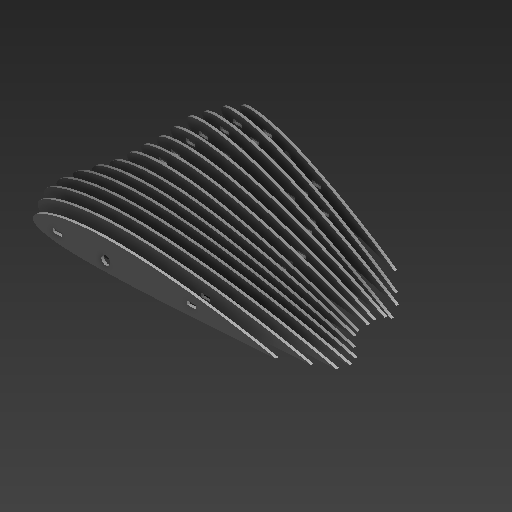
# Autodesk Inventor part: blade_all_sections
Saved by Autodesk Inventor 2027 (Build 310192000, 192)
## iProperties
Created: 2026-04-25
Part Number: blade_all_sections
Material: Generic
Document SubType Name: Modeling
Designer: charl
Density: 1 g/cm^3
Appearance: Default
Author: charl
Autodesk Inventor part; units mm, degrees
(part 1 of 6)
ref_plane "YZ Plane" through (0, 0, 0) normal (1, 0, 0) x (0, 1, 0)
ref_plane "XZ Plane" through (0, 0, 0) normal (0, 1, 0) x (-1, 0, 0)
ref_plane "XY Plane" through (0, 0, 0) normal (0, 0, 1) x (1, 0, 0)
sketch "Template_1mm" plane through (0, 0, 0) normal (0, 0, 1) x (1, 0, 0)
  spline S0 degree 4 poles (1, 0) (0.9999, 0) (0.9991, 0.0002) (0.9979, 0.0004) (0.9958, 0.0009) (0.9936, 0.0014) (0.991, 0.0019) (0.9878, 0.0026) (0.9842, 0.0033) (0.9801, 0.0042) (0.9755, 0.0051) (0.9705, 0.0062) (0.965, 0.0073) (0.959, 0.0085) (0.9526, 0.0098) (0.9457, 0.0112) (0.9384, 0.0126) (0.9307, 0.0141) (0.9226, 0.0157) (0.914, 0.0173) (0.905, 0.019) (0.8957, 0.0207) (0.8859, 0.0225) (0.8758, 0.0243) (0.8652, 0.0261) (0.8544, 0.028) (0.8431, 0.0299) (0.8315, 0.0319) (0.8196, 0.0338) (0.8074, 0.0358) (0.7949, 0.0378) (0.7821, 0.0398) (0.769, 0.0418) (0.7556, 0.0437) (0.742, 0.0457) (0.7281, 0.0477) (0.714, 0.0496) (0.6997, 0.0515) (0.6852, 0.0534) (0.6705, 0.0553) (0.6556, 0.0571) (0.6405, 0.0589) (0.6254, 0.0606) (0.6101, 0.0623) (0.5946, 0.0639) (0.5791, 0.0655) (0.5635, 0.067) (0.5478, 0.0684) (0.5321, 0.0698) (0.5164, 0.0711) (0.5006, 0.0723) (0.4848, 0.0735) (0.469, 0.0745) (0.4533, 0.0755) (0.4376, 0.0763) (0.4219, 0.0771) (0.4064, 0.0778) (0.3908, 0.0783) (0.3754, 0.0788) (0.36, 0.0791) (0.3448, 0.0792) (0.3297, 0.0792) (0.3148, 0.0791) (0.3001, 0.0788) (0.2855, 0.0784) (0.2712, 0.0778) (0.2571, 0.0771) (0.2433, 0.0763) (0.2298, 0.0753) (0.2165, 0.0742) (0.2035, 0.073) (0.1908, 0.0716) (0.1784, 0.0701) (0.1663, 0.0685) (0.1546, 0.0668) (0.1433, 0.065) (0.1323, 0.0631) (0.1217, 0.061) (0.1114, 0.0589) (0.1016, 0.0567) (0.0922, 0.0544) (0.0832, 0.052) (0.0746, 0.0496) (0.0665, 0.0471) (0.0588, 0.0445) (0.0515, 0.0419) (0.0447, 0.0393) (0.0384, 0.0366) (0.0325, 0.0338) (0.0271, 0.0311) (0.0222, 0.0283) (0.0178, 0.0255) (0.0138, 0.0227) (0.0103, 0.0199) (0.0074, 0.0171) (0.0049, 0.0142) (0.0029, 0.0114) (0.0014, 0.0085) (0.0004, 0.0057) (-0.0001, 0.0028) (-0.0001, 0) (0.0004, -0.0028) (0.0015, -0.0055) (0.003, -0.0081) (0.005, -0.0106) (0.0075, -0.013) (0.0105, -0.0153) (0.014, -0.0175) (0.0179, -0.0196) (0.0222, -0.0216) (0.0271, -0.0235) (0.0323, -0.0254) (0.0381, -0.0271) (0.0442, -0.0287) (0.0508, -0.0303) (0.0579, -0.0317) (0.0653, -0.0331) (0.0732, -0.0343) (0.0815, -0.0355) (0.0901, -0.0366) (0.0992, -0.0376) (0.1086, -0.0384) (0.1184, -0.0392) (0.1286, -0.0399) (0.1391, -0.0405) (0.15, -0.041) (0.1612, -0.0415) (0.1727, -0.0418) (0.1845, -0.0421) (0.1966, -0.0423) (0.209, -0.0424) (0.2217, -0.0424) (0.2347, -0.0423) (0.2479, -0.0422) (0.2613, -0.0421) (0.275, -0.0418) (0.2889, -0.0415) (0.303, -0.0412) (0.3173, -0.0408) (0.3318, -0.0404) (0.3464, -0.0399) (0.3612, -0.0394) (0.3761, -0.0389) (0.3911, -0.0383) (0.4063, -0.0378) (0.4217, -0.0371) (0.4371, -0.0365) (0.4526, -0.0358) (0.4682, -0.035) (0.4838, -0.0342) (0.4994, -0.0334) (0.515, -0.0326) (0.5306, -0.0317) (0.5462, -0.0308) (0.5618, -0.0299) (0.5772, -0.029) (0.5927, -0.0281) (0.608, -0.0271) (0.6232, -0.0262) (0.6383, -0.0252) (0.6533, -0.0243) (0.6681, -0.0233) (0.6828, -0.0224) (0.6973, -0.0214) (0.7116, -0.0205) (0.7257, -0.0195) (0.7395, -0.0186) (0.7532, -0.0177) (0.7666, -0.0168) (0.7797, -0.0159) (0.7926, -0.015) (0.8052, -0.0141) (0.8175, -0.0133) (0.8294, -0.0125) (0.8411, -0.0117) (0.8524, -0.0109) (0.8634, -0.0101) (0.874, -0.0093) (0.8842, -0.0086) (0.8941, -0.0079) (0.9036, -0.0072) (0.9126, -0.0065) (0.9213, -0.0059) (0.9296, -0.0053) (0.9374, -0.0047) (0.9448, -0.0042) (0.9518, -0.0037) (0.9583, -0.0032) (0.9643, -0.0027) (0.9699, -0.0023) (0.9751, -0.0019) (0.9797, -0.0016) (0.9839, -0.0012) (0.9876, -0.001) (0.9908, -0.0007) (0.9935, -0.0005) (0.9957, -0.0003) (0.9979, -0.0002) (0.9991, -0.0001) (0.9998, 0) (1, 0) knots 0 0 0 0 0 0.003306 0.005253 0.00752 0.010062 0.01285 0.015861 0.019079 0.022488 0.026078 0.029837 0.033757 0.037828 0.042045 0.046398 0.050884 0.055494 0.060224 0.065069 0.070023 0.075082 0.080241 0.085495 0.090841 0.096274 0.101791 0.107386 0.113057 0.118799 0.124609 0.130484 0.136419 0.142412 0.148458 0.154554 0.160697 0.166884 0.17311 0.179374 0.185671 0.191998 0.198352 0.20473 0.211128 0.217543 0.223972 0.230412 0.23686 0.243312 0.249765 0.256217 0.262663 0.2691 0.275526 0.281941 0.288345 0.294734 0.301105 0.307451 0.313767 0.320049 0.326294 0.332498 0.338659 0.344773 0.350837 0.356848 0.362801 0.368695 0.374525 0.380288 0.38598 0.391599 0.39714 0.4026 0.407976 0.413263 0.418458 0.423557 0.428556 0.433452 0.438241 0.442917 0.447478 0.451919 0.456236 0.460425 0.464482 0.468403 0.472185 0.475825 0.479322 0.482675 0.485889 0.48897 0.49193 0.494788 0.497572 0.50031 0.503032 0.505769 0.508552 0.511409 0.514365 0.517441 0.520647 0.523991 0.527474 0.531098 0.534861 0.538758 0.542789 0.546947 0.551231 0.555634 0.560154 0.564786 0.569527 0.574371 0.579315 0.584356 0.58949 0.594712 0.60002 0.605409 0.610877 0.61642 0.622034 0.627716 0.633463 0.639271 0.645138 0.651061 0.657035 0.663059 0.669128 0.675241 0.681393 0.687582 0.693804 0.700057 0.706341 0.712655 0.718998 0.725365 0.731751 0.738149 0.744556 0.750969 0.757385 0.7638 0.770211 0.776616 0.783011 0.789393 0.795759 0.802106 0.808429 0.814727 0.820996 0.827232 0.833433 0.839595 0.845714 0.851788 0.857813 0.863785 0.869702 0.875558 0.881352 0.887078 0.892735 0.898316 0.90382 0.909242 0.914577 0.919822 0.924972 0.930023 0.93497 0.939808 0.944533 0.949139 0.95362 0.95797 0.962183 0.966252 0.970169 0.973927 0.977515 0.980924 0.984141 0.987151 0.989939 0.99248 0.994747 0.996694 1 1 1 1 1
  point P0 (0, 0)
  point P1 (0.999, 0.0002)
  point P2 (0.9978, 0.0005)
  point P3 (0.9961, 0.0008)
  point P4 (0.9939, 0.0013)
  point P5 (0.9912, 0.0019)
  point P6 (0.9881, 0.0025)
  point P7 (0.9844, 0.0033)
  point P8 (0.9803, 0.0041)
  point P9 (0.9758, 0.0051)
  point P10 (0.9707, 0.0061)
  point P11 (0.9652, 0.0073)
  point P12 (0.9592, 0.0085)
  point P13 (0.9528, 0.0097)
  point P14 (0.946, 0.0111)
  point P15 (0.9387, 0.0125)
  point P16 (0.9309, 0.014)
  point P17 (0.9228, 0.0156)
  point P18 (0.9142, 0.0172)
  point P19 (0.9052, 0.0189)
  point P20 (0.8959, 0.0206)
  point P21 (0.8861, 0.0224)
  point P22 (0.8759, 0.0242)
  point P23 (0.8654, 0.0261)
  point P24 (0.8545, 0.028)
  point P25 (0.8433, 0.0299)
  point P26 (0.8317, 0.0318)
  point P27 (0.8198, 0.0338)
  point P28 (0.8076, 0.0358)
  point P29 (0.795, 0.0378)
  point P30 (0.7822, 0.0397)
  point P31 (0.7691, 0.0417)
  point P32 (0.7557, 0.0437)
  point P33 (0.7421, 0.0457)
  point P34 (0.7282, 0.0476)
  point P35 (0.7141, 0.0496)
  point P36 (0.6998, 0.0515)
  point P37 (0.6853, 0.0534)
  point P38 (0.6705, 0.0553)
  point P39 (0.6557, 0.0571)
  point P40 (0.6406, 0.0589)
  point P41 (0.6254, 0.0606)
  point P42 (0.6101, 0.0623)
  point P43 (0.5947, 0.0639)
  point P44 (0.5792, 0.0655)
  point P45 (0.5635, 0.067)
  point P46 (0.5479, 0.0684)
  point P47 (0.5321, 0.0698)
  point P48 (0.5164, 0.0711)
  point P49 (0.5006, 0.0723)
  point P50 (0.4848, 0.0734)
  point P51 (0.469, 0.0745)
  point P52 (0.4533, 0.0754)
  point P53 (0.4376, 0.0763)
  point P54 (0.4219, 0.0771)
  point P55 (0.4064, 0.0778)
  point P56 (0.3908, 0.0783)
  point P57 (0.3753, 0.0787)
  point P58 (0.3599, 0.079)
  point P59 (0.3447, 0.0792)
  point P60 (0.3296, 0.0792)
  point P61 (0.3147, 0.0791)
  point P62 (0.2999, 0.0788)
  point P63 (0.2854, 0.0784)
  point P64 (0.2711, 0.0778)
  point P65 (0.257, 0.0771)
  point P66 (0.2432, 0.0763)
  point P67 (0.2296, 0.0753)
  point P68 (0.2163, 0.0742)
  point P69 (0.2033, 0.0729)
  point P70 (0.1906, 0.0716)
  point P71 (0.1782, 0.0701)
  point P72 (0.1662, 0.0685)
  point P73 (0.1544, 0.0668)
  point P74 (0.1431, 0.0649)
  point P75 (0.1321, 0.063)
  point P76 (0.1215, 0.061)
  point P77 (0.1112, 0.0588)
  point P78 (0.1014, 0.0566)
  point P79 (0.092, 0.0543)
  point P80 (0.083, 0.052)
  point P81 (0.0744, 0.0495)
  point P82 (0.0663, 0.047)
  point P83 (0.0586, 0.0444)
  point P84 (0.0513, 0.0418)
  point P85 (0.0445, 0.0391)
  point P86 (0.0382, 0.0364)
  point P87 (0.0323, 0.0337)
  point P88 (0.027, 0.0309)
  point P89 (0.0221, 0.0282)
  point P90 (0.0176, 0.0253)
  point P91 (0.0137, 0.0225)
  point P92 (0.0102, 0.0197)
  point P93 (0.0073, 0.0169)
  point P94 (0.0048, 0.014)
  point P95 (0.0029, 0.0112)
  point P96 (0.0014, 0.0084)
  point P97 (0.0004, 0.0056)
  point P98 (0, 0.0028)
  point P99 (0, 0)
  point P100 (0.0005, -0.0027)
  point P101 (0.0015, -0.0054)
  point P102 (0.003, -0.008)
  point P103 (0.005, -0.0104)
  point P104 (0.0075, -0.0128)
  point P105 (0.0104, -0.0151)
  point P106 (0.0138, -0.0173)
  point P107 (0.0177, -0.0195)
  point P108 (0.0221, -0.0215)
  point P109 (0.0269, -0.0234)
  point P110 (0.0322, -0.0252)
  point P111 (0.0379, -0.027)
  point P112 (0.044, -0.0286)
  point P113 (0.0506, -0.0302)
  point P114 (0.0577, -0.0317)
  point P115 (0.0651, -0.033)
  point P116 (0.073, -0.0343)
  point P117 (0.0813, -0.0355)
  point P118 (0.0899, -0.0365)
  point P119 (0.099, -0.0375)
  point P120 (0.1084, -0.0384)
  point P121 (0.1182, -0.0392)
  point P122 (0.1284, -0.0399)
  point P123 (0.1389, -0.0405)
  point P124 (0.1498, -0.041)
  point P125 (0.161, -0.0414)
  point P126 (0.1725, -0.0418)
  point P127 (0.1844, -0.0421)
  point P128 (0.1965, -0.0422)
  point P129 (0.2089, -0.0423)
  point P130 (0.2216, -0.0424)
  point P131 (0.2346, -0.0423)
  point P132 (0.2478, -0.0422)
  point P133 (0.2612, -0.0421)
  point P134 (0.2749, -0.0418)
  point P135 (0.2888, -0.0415)
  point P136 (0.3029, -0.0412)
  point P137 (0.3172, -0.0408)
  point P138 (0.3317, -0.0404)
  point P139 (0.3463, -0.0399)
  point P140 (0.3611, -0.0394)
  point P141 (0.376, -0.0389)
  point P142 (0.3911, -0.0383)
  point P143 (0.4063, -0.0378)
  point P144 (0.4216, -0.0371)
  point P145 (0.4371, -0.0365)
  point P146 (0.4526, -0.0358)
  point P147 (0.4682, -0.035)
  point P148 (0.4838, -0.0342)
  point P149 (0.4994, -0.0334)
  point P150 (0.515, -0.0326)
  point P151 (0.5307, -0.0317)
  point P152 (0.5462, -0.0308)
  point P153 (0.5618, -0.0299)
  point P154 (0.5773, -0.029)
  point P155 (0.5927, -0.0281)
  point P156 (0.608, -0.0271)
  point P157 (0.6233, -0.0262)
  point P158 (0.6384, -0.0252)
  point P159 (0.6534, -0.0243)
  point P160 (0.6682, -0.0233)
  point P161 (0.6829, -0.0224)
  point P162 (0.6974, -0.0214)
  point P163 (0.7117, -0.0205)
  point P164 (0.7258, -0.0195)
  point P165 (0.7397, -0.0186)
  point P166 (0.7533, -0.0177)
  point P167 (0.7667, -0.0168)
  point P168 (0.7799, -0.0159)
  point P169 (0.7927, -0.015)
  point P170 (0.8053, -0.0141)
  point P171 (0.8176, -0.0133)
  point P172 (0.8296, -0.0125)
  point P173 (0.8413, -0.0116)
  point P174 (0.8526, -0.0108)
  point P175 (0.8636, -0.0101)
  point P176 (0.8742, -0.0093)
  point P177 (0.8844, -0.0086)
  point P178 (0.8943, -0.0079)
  point P179 (0.9038, -0.0072)
  point P180 (0.9129, -0.0065)
  point P181 (0.9215, -0.0059)
  point P182 (0.9298, -0.0053)
  point P183 (0.9376, -0.0047)
  point P184 (0.945, -0.0042)
  point P185 (0.952, -0.0037)
  point P186 (0.9585, -0.0032)
  point P187 (0.9646, -0.0027)
  point P188 (0.9702, -0.0023)
  point P189 (0.9753, -0.0019)
  point P190 (0.98, -0.0015)
  point P191 (0.9841, -0.0012)
  point P192 (0.9878, -0.0009)
  point P193 (0.9911, -0.0007)
  point P194 (0.9938, -0.0005)
  point P195 (0.996, -0.0003)
  point P196 (0.9978, -0.0002)
  point P197 (0.999, -0.0001)
  point P198 (0.9998, 0)
  constraints: 201 other
sketch "S01_282p7" plane through (0, 0, 0) normal (0, 0, 1) x (1, 0, 0)
  spline S0 degree 4 poles (197.89, 0) (197.8478, 0.0089) (197.6412, 0.0535) (197.2945, 0.127) (196.7094, 0.2515) (196.0938, 0.3827) (195.3375, 0.5419) (194.4468, 0.7301) (193.42, 0.9446) (192.2596, 1.1868) (190.9662, 1.454) (189.5407, 1.7472) (187.9852, 2.0644) (186.3002, 2.405) (184.4884, 2.7686) (182.5503, 3.1528) (180.4886, 3.5578) (178.305, 3.9817) (176.0014, 4.4244) (173.5799, 4.8834) (171.0432, 5.3581) (168.3934, 5.8471) (165.6328, 6.3494) (162.7648, 6.8637) (159.791, 7.3884) (156.7155, 7.9219) (153.54, 8.464) (150.2688, 9.0122) (146.9036, 9.5662) (143.4493, 10.1234) (139.9076, 10.6839) (136.2831, 11.2451) (132.5788, 11.8067) (128.7985, 12.3666) (124.9455, 12.924) (121.0243, 13.4777) (117.0377, 14.0257) (112.9904, 14.5674) (108.8863, 15.1011) (104.729, 15.6259) (100.5229, 16.1401) (96.2719, 16.6428) (91.9805, 17.1328) (87.6529, 17.6088) (83.2929, 18.069) (78.9059, 18.5129) (74.4948, 18.9397) (70.0653, 19.3466) (65.6209, 19.7344) (61.1668, 20.1005) (56.7065, 20.4449) (52.2457, 20.7659) (47.7877, 21.0617) (43.3377, 21.3337) (38.8997, 21.5782) (34.4748, 21.7965) (30.0745, 21.9858) (25.679, 22.1479) (21.302, 22.268) (16.9599, 22.3503) (12.6537, 22.3924) (8.3912, 22.3942) (4.1763, 22.3569) (0.0143, 22.2781) (-4.0915, 22.161) (-8.1355, 22.0027) (-12.1145, 21.806) (-16.0234, 21.5697) (-19.8589, 21.2958) (-23.6162, 20.9836) (-27.292, 20.6351) (-30.8818, 20.2504) (-34.3822, 19.8314) (-37.7896, 19.378) (-41.1001, 18.8929) (-44.3103, 18.3764) (-47.4177, 17.8306) (-50.4179, 17.2562) (-53.3089, 16.6561) (-56.0871, 16.0307) (-58.7501, 15.3815) (-61.2951, 14.7119) (-63.7196, 14.0219) (-66.0212, 13.3139) (-68.1983, 12.5902) (-70.248, 11.8516) (-72.169, 11.1005) (-73.9594, 10.3386) (-75.6179, 9.5672) (-77.1424, 8.7878) (-78.5328, 8.0024) (-79.7874, 7.2122) (-80.905, 6.4176) (-81.8865, 5.6212) (-82.7292, 4.8217) (-83.4343, 4.0206) (-84.0005, 3.2181) (-84.4265, 2.4131) (-84.7091, 1.6061) (-84.8481, 0.8003) (-84.8395, -0.0029) (-84.6887, -0.7919) (-84.3938, -1.5543) (-83.9585, -2.2892) (-83.3855, -2.9949) (-82.6774, -3.672) (-81.836, -4.3207) (-80.8623, -4.9429) (-79.7576, -5.5386) (-78.5226, -6.1081) (-77.1584, -6.6512) (-75.6665, -7.1679) (-74.048, -7.6582) (-72.3049, -8.1218) (-70.4387, -8.559) (-68.4516, -8.9688) (-66.3451, -9.3525) (-64.122, -9.7084) (-61.7838, -10.0379) (-59.3335, -10.3407) (-56.7729, -10.6165) (-54.1052, -10.8651) (-51.3323, -11.0888) (-48.4575, -11.2848) (-45.4833, -11.4565) (-42.4121, -11.602) (-39.2476, -11.7234) (-35.9922, -11.8211) (-32.6493, -11.8942) (-29.2217, -11.9463) (-25.7127, -11.9747) (-22.1257, -11.9838) (-18.464, -11.9717) (-14.7302, -11.941) (-10.929, -11.8928) (-7.0625, -11.8268) (-3.1355, -11.7458) (0.8493, -11.6499) (4.888, -11.5404) (8.977, -11.4191) (13.1124, -11.2874) (17.2906, -11.1451) (21.5102, -10.9956) (25.7647, -10.837) (30.0612, -10.676) (34.4055, -10.4993) (38.7678, -10.3113) (43.1533, -10.1102) (47.5518, -9.8987) (51.9606, -9.6775) (56.375, -9.4478) (60.7901, -9.2098) (65.2023, -8.9656) (69.607, -8.7144) (74.0002, -8.4593) (78.3772, -8.1988) (82.734, -7.936) (87.066, -7.6701) (91.3697, -7.4015) (95.6399, -7.1328) (99.8729, -6.8629) (104.0645, -6.5924) (108.2108, -6.3235) (112.3068, -6.0547) (116.3497, -5.7881) (120.3344, -5.5234) (124.2575, -5.2608) (128.1148, -5.0011) (131.9031, -4.7449) (135.6174, -4.4924) (139.255, -4.2434) (142.812, -3.9985) (146.2846, -3.759) (149.6692, -3.5233) (152.963, -3.2936) (156.162, -3.0687) (159.2633, -2.8504) (162.2636, -2.637) (165.1601, -2.4307) (167.9493, -2.2306) (170.6291, -2.0375) (173.1959, -1.851) (175.648, -1.6728) (177.982, -1.5013) (180.196, -1.3384) (182.2877, -1.1837) (184.2548, -1.0368) (186.0952, -0.8993) (187.8074, -0.7709) (189.389, -0.6512) (190.8386, -0.5416) (192.1549, -0.4409) (193.336, -0.3512) (194.3812, -0.2707) (195.2888, -0.201) (196.0589, -0.1419) (196.6867, -0.0929) (197.2832, -0.0475) (197.6364, -0.0194) (197.8469, -0.0032) (197.89, 0) knots 0 0 0 0 0 0.003306 0.005253 0.00752 0.010062 0.01285 0.015861 0.019079 0.022488 0.026078 0.029837 0.033757 0.037828 0.042045 0.046398 0.050884 0.055494 0.060224 0.065069 0.070023 0.075082 0.080241 0.085495 0.090841 0.096274 0.101791 0.107386 0.113057 0.118799 0.124609 0.130484 0.136419 0.142412 0.148458 0.154554 0.160697 0.166884 0.17311 0.179374 0.185671 0.191998 0.198352 0.20473 0.211128 0.217543 0.223972 0.230412 0.23686 0.243312 0.249765 0.256217 0.262663 0.2691 0.275526 0.281941 0.288345 0.294734 0.301105 0.307451 0.313767 0.320049 0.326294 0.332498 0.338659 0.344773 0.350837 0.356848 0.362801 0.368695 0.374525 0.380288 0.38598 0.391599 0.39714 0.4026 0.407976 0.413263 0.418458 0.423557 0.428556 0.433452 0.438241 0.442917 0.447478 0.451919 0.456236 0.460425 0.464482 0.468403 0.472185 0.475825 0.479322 0.482675 0.485889 0.48897 0.49193 0.494788 0.497572 0.50031 0.503032 0.505769 0.508552 0.511409 0.514365 0.517441 0.520647 0.523991 0.527474 0.531098 0.534861 0.538758 0.542789 0.546947 0.551231 0.555634 0.560154 0.564786 0.569527 0.574371 0.579315 0.584356 0.58949 0.594712 0.60002 0.605409 0.610877 0.61642 0.622034 0.627716 0.633463 0.639271 0.645138 0.651061 0.657035 0.663059 0.669128 0.675241 0.681393 0.687582 0.693804 0.700057 0.706341 0.712655 0.718998 0.725365 0.731751 0.738149 0.744556 0.750969 0.757385 0.7638 0.770211 0.776616 0.783011 0.789393 0.795759 0.802106 0.808429 0.814727 0.820996 0.827232 0.833433 0.839595 0.845714 0.851788 0.857813 0.863785 0.869702 0.875558 0.881352 0.887078 0.892735 0.898316 0.90382 0.909242 0.914577 0.919822 0.924972 0.930023 0.93497 0.939808 0.944533 0.949139 0.95362 0.95797 0.962183 0.966252 0.970169 0.973927 0.977515 0.980924 0.984141 0.987151 0.989939 0.99248 0.994747 0.996694 1 1 1 1 1
  circle A0 centre (0, 0) radius 5.15
  line L0 (-51.44, -2.1) -> (-61.64, -2.1)
  line L1 (-61.64, -2.1) -> (-61.64, 2.1)
  line L2 (-61.64, 2.1) -> (-51.44, 2.1)
  line L3 (-51.44, 2.1) -> (-51.44, -2.1)
  line L4 (-51.44, -2.1) -> (-61.64, 2.1) construction
  line L5 (-61.64, -2.1) -> (-51.44, 2.1) construction
  line L6 (105.1, 7.1) -> (94.9, 7.1)
  line L7 (94.9, 7.1) -> (94.9, 2.9)
  line L8 (94.9, 2.9) -> (105.1, 2.9)
  line L9 (105.1, 2.9) -> (105.1, 7.1)
  line L10 (105.1, 7.1) -> (94.9, 2.9) construction
  line L11 (94.9, 7.1) -> (105.1, 2.9) construction
  point P0 (197.6138, 0.0591)
  point P1 (197.2686, 0.1326)
  point P2 (196.7861, 0.2352)
  point P3 (196.1664, 0.3669)
  point P4 (195.4102, 0.5267)
  point P5 (194.518, 0.7147)
  point P6 (193.4906, 0.9298)
  point P7 (192.3293, 1.1718)
  point P8 (191.0351, 1.4395)
  point P9 (189.6089, 1.7327)
  point P10 (188.0523, 2.0501)
  point P11 (186.3666, 2.3911)
  point P12 (184.5536, 2.7546)
  point P13 (182.6146, 3.1394)
  point P14 (180.5517, 3.5445)
  point P15 (178.367, 3.9688)
  point P16 (176.0622, 4.4115)
  point P17 (173.6394, 4.8709)
  point P18 (171.1013, 5.3459)
  point P19 (168.4502, 5.8352)
  point P20 (165.6882, 6.3379)
  point P21 (162.8185, 6.8524)
  point P22 (159.8434, 7.3773)
  point P23 (156.7662, 7.9114)
  point P24 (153.5892, 8.4536)
  point P25 (150.3161, 9.0023)
  point P26 (146.9494, 9.5564)
  point P27 (143.4931, 10.1142)
  point P28 (139.9498, 10.6748)
  point P29 (136.3233, 11.2365)
  point P30 (132.6171, 11.7982)
  point P31 (128.8349, 12.3585)
  point P32 (124.98, 12.9163)
  point P33 (121.0567, 13.4701)
  point P34 (117.068, 14.0185)
  point P35 (113.0187, 14.5605)
  point P36 (108.9124, 15.0945)
  point P37 (104.7531, 15.6195)
  point P38 (100.5448, 16.134)
  point P39 (96.2916, 16.6369)
  point P40 (91.9979, 17.1271)
  point P41 (87.6681, 17.6032)
  point P42 (83.306, 18.0637)
  point P43 (78.9166, 18.5078)
  point P44 (74.5033, 18.9344)
  point P45 (70.0714, 19.3418)
  point P46 (65.6248, 19.7294)
  point P47 (61.1684, 20.0957)
  point P48 (56.7059, 20.4401)
  point P49 (52.2427, 20.7609)
  point P50 (47.7825, 21.0572)
  point P51 (43.3303, 21.3286)
  point P52 (38.8902, 21.5734)
  point P53 (34.4671, 21.7911)
  point P54 (30.0651, 21.9805)
  point P55 (25.668, 22.1397)
  point P56 (21.2865, 22.2606)
  point P57 (16.9394, 22.3423)
  point P58 (12.631, 22.3842)
  point P59 (8.3662, 22.3859)
  point P60 (4.1495, 22.3477)
  point P61 (-0.0147, 22.2691)
  point P62 (-4.1223, 22.151)
  point P63 (-8.1683, 21.9926)
  point P64 (-12.149, 21.795)
  point P65 (-16.0599, 21.5584)
  point P66 (-19.897, 21.2836)
  point P67 (-23.6561, 20.971)
  point P68 (-27.3334, 20.6216)
  point P69 (-30.9248, 20.2362)
  point P70 (-34.4266, 19.8161)
  point P71 (-37.8354, 19.3621)
  point P72 (-41.1473, 18.8759)
  point P73 (-44.3587, 18.3585)
  point P74 (-47.467, 17.8115)
  point P75 (-50.4685, 17.2362)
  point P76 (-53.3602, 16.6346)
  point P77 (-56.1391, 16.0079)
  point P78 (-58.8027, 15.3577)
  point P79 (-61.3482, 14.6863)
  point P80 (-63.7729, 13.9948)
  point P81 (-66.0746, 13.2852)
  point P82 (-68.2514, 12.5595)
  point P83 (-70.3007, 11.8191)
  point P84 (-72.2208, 11.066)
  point P85 (-74.01, 10.3019)
  point P86 (-75.6666, 9.5281)
  point P87 (-77.189, 8.7465)
  point P88 (-78.5762, 7.9586)
  point P89 (-79.8266, 7.1659)
  point P90 (-80.9393, 6.3695)
  point P91 (-81.9137, 5.5712)
  point P92 (-82.7486, 4.7714)
  point P93 (-83.4437, 3.9717)
  point P94 (-83.9987, 3.173)
  point P95 (-84.4128, 2.3758)
  point P96 (-84.6859, 1.5809)
  point P97 (-84.8185, 0.7887)
  point P98 (-84.81, 0)
  point P99 (-84.6621, -0.7749)
  point P100 (-84.3761, -1.5252)
  point P101 (-83.9526, -2.2506)
  point P102 (-83.3923, -2.9511)
  point P103 (-82.6957, -3.6265)
  point P104 (-81.864, -4.2761)
  point P105 (-80.898, -4.9003)
  point P106 (-79.7991, -5.4988)
  point P107 (-78.5685, -6.0713)
  point P108 (-77.2076, -6.6174)
  point P109 (-75.7181, -7.137)
  point P110 (-74.1013, -7.6301)
  point P111 (-72.3593, -8.0962)
  point P112 (-70.4938, -8.5356)
  point P113 (-68.507, -8.9477)
  point P114 (-66.4006, -9.3331)
  point P115 (-64.1771, -9.691)
  point P116 (-61.8386, -10.022)
  point P117 (-59.3876, -10.3262)
  point P118 (-56.8264, -10.6032)
  point P119 (-54.1577, -10.8534)
  point P120 (-51.3838, -11.0776)
  point P121 (-48.5079, -11.2752)
  point P122 (-45.5325, -11.4474)
  point P123 (-42.4601, -11.5941)
  point P124 (-39.2942, -11.7162)
  point P125 (-36.0375, -11.8143)
  point P126 (-32.6931, -11.8887)
  point P127 (-29.264, -11.9407)
  point P128 (-25.7534, -11.9704)
  point P129 (-22.1648, -11.9794)
  point P130 (-18.5013, -11.9681)
  point P131 (-14.766, -11.9379)
  point P132 (-10.9628, -11.8898)
  point P133 (-7.0946, -11.8245)
  point P134 (-3.1657, -11.7436)
  point P135 (0.821, -11.6481)
  point P136 (4.8616, -11.539)
  point P137 (8.9525, -11.418)
  point P138 (13.0899, -11.2862)
  point P139 (17.2699, -11.1446)
  point P140 (21.4889, -10.9948)
  point P141 (25.7429, -10.8376)
  point P142 (30.0422, -10.6739)
  point P143 (34.389, -10.4978)
  point P144 (38.7579, -10.3092)
  point P145 (43.1454, -10.1085)
  point P146 (47.5465, -9.897)
  point P147 (51.9574, -9.676)
  point P148 (56.3741, -9.4461)
  point P149 (60.7915, -9.2084)
  point P150 (65.2059, -8.9639)
  point P151 (69.6129, -8.7131)
  point P152 (74.0083, -8.4575)
  point P153 (78.3876, -8.1975)
  point P154 (82.7466, -7.9343)
  point P155 (87.0809, -7.6682)
  point P156 (91.3867, -7.4)
  point P157 (95.6592, -7.1308)
  point P158 (99.8943, -6.8608)
  point P159 (104.0882, -6.5906)
  point P160 (108.2365, -6.3212)
  point P161 (112.3348, -6.0526)
  point P162 (116.3797, -5.7857)
  point P163 (120.3666, -5.5208)
  point P164 (124.2916, -5.2582)
  point P165 (128.151, -4.9984)
  point P166 (131.9412, -4.742)
  point P167 (135.6576, -4.4893)
  point P168 (139.297, -4.2402)
  point P169 (142.8559, -3.9954)
  point P170 (146.3303, -3.7554)
  point P171 (149.7168, -3.5199)
  point P172 (153.0122, -3.2898)
  point P173 (156.213, -3.065)
  point P174 (159.3159, -2.8462)
  point P175 (162.3179, -2.6331)
  point P176 (165.2158, -2.4264)
  point P177 (168.0066, -2.2263)
  point P178 (170.6878, -2.0329)
  point P179 (173.2561, -1.8466)
  point P180 (175.7094, -1.6679)
  point P181 (178.0447, -1.4966)
  point P182 (180.26, -1.3335)
  point P183 (182.3528, -1.1786)
  point P184 (184.321, -1.0319)
  point P185 (186.1625, -0.8942)
  point P186 (187.8756, -0.7656)
  point P187 (189.4582, -0.646)
  point P188 (190.9087, -0.536)
  point P189 (192.2258, -0.4356)
  point P190 (193.4078, -0.3455)
  point P191 (194.4538, -0.2652)
  point P192 (195.3627, -0.1953)
  point P193 (196.133, -0.136)
  point P194 (196.7649, -0.0871)
  point P195 (197.2568, -0.0492)
  point P196 (197.6084, -0.0218)
  point P197 (197.8196, -0.0054)
  point P198 (-84.81, 0)
  point P199 (-56.54, 0)
  dimension "d0" = 10.3
  dimension "d1" = 84.81
  dimension "d32" = 10.2
  dimension "d33" = 4.2
  dimension "d36" = -56.54
  dimension "d184" = 10.2
  dimension "d185" = 4.2
  dimension "d186" = 5
  dimension "d187" = 100
  constraints: 24 end point, 4 midpoint, 4 parallel, 2 horizontal, 2 perpendicular, 1 centre point, 202 other
  measures "d0" diameter of A0
  measures "d1" distance of A0.centre point (-84.81, 0)
  measures "d32" distance of L1.end L2.end
  measures "d33" distance of L0.end L1.end
  measures "d36" distance of A0.centre point (-56.54, 0)
  measures "d184" distance of L8.end L7.end
  measures "d185" distance of L7.end L6.end
  measures "d186" vertical distance of A0.centre point (100, 5)
  measures "d187" horizontal distance of point (100, 5) A0.centre
sketch "S02_317p9" plane through (0, 0, 0) normal (0, 0, 1) x (1, 0, 0)
  spline S0 degree 4 poles (222.5219, -1.9031) (222.4744, -1.8927) (222.2427, -1.8405) (221.8535, -1.7545) (221.1967, -1.609) (220.5057, -1.4555) (219.6568, -1.2692) (218.6571, -1.049) (217.5046, -0.7979) (216.2021, -0.5144) (214.7502, -0.2016) (213.1501, 0.1419) (211.404, 0.5135) (209.5126, 0.9127) (207.4788, 1.339) (205.3031, 1.7897) (202.9887, 2.265) (200.5374, 2.7626) (197.9513, 3.2826) (195.2328, 3.8219) (192.3849, 4.3801) (189.41, 4.9554) (186.3106, 5.5469) (183.0905, 6.1527) (179.7516, 6.7714) (176.2985, 7.4008) (172.7329, 8.041) (169.0598, 8.6889) (165.2811, 9.3442) (161.4022, 10.0039) (157.425, 10.6683) (153.3548, 11.3342) (149.1947, 12.0013) (144.9493, 12.6672) (140.622, 13.3312) (136.2182, 13.9914) (131.7405, 14.6459) (127.1947, 15.2941) (122.5849, 15.9336) (117.9151, 16.5638) (113.1905, 17.1824) (108.4152, 17.7885) (103.5943, 18.3808) (98.7327, 18.9577) (93.8344, 19.5171) (88.9055, 20.0585) (83.9495, 20.5808) (78.9726, 21.0809) (73.9786, 21.5597) (68.9737, 22.0142) (63.9616, 22.4444) (58.9485, 22.8483) (53.9385, 23.2238) (48.9372, 23.5724) (43.9492, 23.89) (38.9755, 24.1781) (34.0294, 24.4332) (29.0883, 24.6577) (24.1677, 24.8349) (19.2858, 24.9692) (14.4441, 25.058) (9.651, 25.1009) (4.9112, 25.0995) (0.2303, 25.051) (-4.3877, 24.9588) (-8.9365, 24.8197) (-13.4127, 24.6367) (-17.8105, 24.4086) (-22.126, 24.1376) (-26.3539, 23.8226) (-30.4906, 23.466) (-34.531, 23.068) (-38.4711, 22.6305) (-42.307, 22.1534) (-46.0343, 21.6398) (-49.649, 21.0899) (-53.1484, 20.5061) (-56.5276, 19.889) (-59.7842, 19.242) (-62.9142, 18.5654) (-65.9149, 17.8611) (-68.7832, 17.1326) (-71.5161, 16.38) (-74.111, 15.606) (-76.5661, 14.8132) (-78.878, 14.0024) (-81.0453, 13.1763) (-83.0659, 12.3368) (-84.9382, 11.4853) (-86.66, 10.6235) (-88.2311, 9.7537) (-89.6493, 8.8772) (-90.9137, 7.9944) (-92.025, 7.1084) (-92.9803, 6.2174) (-93.7809, 5.3235) (-94.4253, 4.4265) (-94.912, 3.5254) (-95.2376, 2.6207) (-95.4016, 1.7159) (-95.3997, 0.8126) (-95.2377, -0.0761) (-94.9135, -0.9361) (-94.431, -1.7668) (-93.7935, -2.5658) (-93.0038, -3.334) (-92.0639, -4.0716) (-90.975, -4.7805) (-89.7385, -5.461) (-88.3552, -6.1132) (-86.8264, -6.7371) (-85.1538, -7.3324) (-83.3386, -7.8994) (-81.383, -8.4374) (-79.2886, -8.9469) (-77.0582, -9.4269) (-74.6932, -9.8786) (-72.1968, -10.3001) (-69.5708, -10.6932) (-66.8184, -11.0573) (-63.9417, -11.392) (-60.9443, -11.6972) (-57.8284, -11.9754) (-54.5976, -12.2234) (-51.2549, -12.4451) (-47.8028, -12.6383) (-44.2456, -12.8052) (-40.5859, -12.9463) (-36.8277, -13.0607) (-32.9739, -13.1522) (-29.0284, -13.218) (-24.995, -13.2627) (-20.8774, -13.2843) (-16.6786, -13.2856) (-12.4038, -13.268) (-8.0553, -13.231) (-3.6388, -13.1777) (0.843, -13.1082) (5.3854, -13.0238) (9.9845, -12.9268) (14.636, -12.8185) (19.3356, -12.6986) (24.0819, -12.5711) (28.8675, -12.4337) (33.7004, -12.294) (38.587, -12.1371) (43.4942, -11.9676) (48.4274, -11.7836) (53.3755, -11.5881) (58.3352, -11.3818) (63.3012, -11.1659) (68.2683, -10.9408) (73.232, -10.7086) (78.1874, -10.4685) (83.1298, -10.2239) (88.0542, -9.9731) (92.9558, -9.7194) (97.8296, -9.4621) (102.6715, -9.2015) (107.4758, -8.9404) (112.2383, -8.6776) (116.9542, -8.4138) (121.6192, -8.1512) (126.2277, -7.8884) (130.7763, -7.6275) (135.2597, -7.3681) (139.6735, -7.1106) (144.0135, -6.8557) (148.2757, -6.6039) (152.4548, -6.3558) (156.5476, -6.1108) (160.5497, -5.8696) (164.4569, -5.6337) (168.265, -5.4012) (171.971, -5.1746) (175.5703, -4.9524) (179.0598, -4.7368) (182.4356, -4.5257) (185.6946, -4.3216) (188.8329, -4.1233) (191.8481, -3.932) (194.7362, -3.747) (197.4952, -3.5702) (200.1214, -3.3998) (202.6126, -3.2379) (204.9661, -3.0841) (207.1795, -2.9378) (209.2503, -2.8009) (211.1768, -2.673) (212.9564, -2.5536) (214.5875, -2.4442) (216.0687, -2.3438) (217.3976, -2.2542) (218.5737, -2.1738) (219.595, -2.1041) (220.4615, -2.045) (221.1679, -1.9959) (221.8391, -1.9506) (222.2365, -1.9225) (222.4734, -1.9063) (222.5219, -1.9031) knots 0 0 0 0 0 0.003306 0.005253 0.00752 0.010062 0.01285 0.015861 0.019079 0.022488 0.026078 0.029837 0.033757 0.037828 0.042045 0.046398 0.050884 0.055494 0.060224 0.065069 0.070023 0.075082 0.080241 0.085495 0.090841 0.096274 0.101791 0.107386 0.113057 0.118799 0.124609 0.130484 0.136419 0.142412 0.148458 0.154554 0.160697 0.166884 0.17311 0.179374 0.185671 0.191998 0.198352 0.20473 0.211128 0.217543 0.223972 0.230412 0.23686 0.243312 0.249765 0.256217 0.262663 0.2691 0.275526 0.281941 0.288345 0.294734 0.301105 0.307451 0.313767 0.320049 0.326294 0.332498 0.338659 0.344773 0.350837 0.356848 0.362801 0.368695 0.374525 0.380288 0.38598 0.391599 0.39714 0.4026 0.407976 0.413263 0.418458 0.423557 0.428556 0.433452 0.438241 0.442917 0.447478 0.451919 0.456236 0.460425 0.464482 0.468403 0.472185 0.475825 0.479322 0.482675 0.485889 0.48897 0.49193 0.494788 0.497572 0.50031 0.503032 0.505769 0.508552 0.511409 0.514365 0.517441 0.520647 0.523991 0.527474 0.531098 0.534861 0.538758 0.542789 0.546947 0.551231 0.555634 0.560154 0.564786 0.569527 0.574371 0.579315 0.584356 0.58949 0.594712 0.60002 0.605409 0.610877 0.61642 0.622034 0.627716 0.633463 0.639271 0.645138 0.651061 0.657035 0.663059 0.669128 0.675241 0.681393 0.687582 0.693804 0.700057 0.706341 0.712655 0.718998 0.725365 0.731751 0.738149 0.744556 0.750969 0.757385 0.7638 0.770211 0.776616 0.783011 0.789393 0.795759 0.802106 0.808429 0.814727 0.820996 0.827232 0.833433 0.839595 0.845714 0.851788 0.857813 0.863785 0.869702 0.875558 0.881352 0.887078 0.892735 0.898316 0.90382 0.909242 0.914577 0.919822 0.924972 0.930023 0.93497 0.939808 0.944533 0.949139 0.95362 0.95797 0.962183 0.966252 0.970169 0.973927 0.977515 0.980924 0.984141 0.987151 0.989939 0.99248 0.994747 0.996694 1 1 1 1 1
  circle A0 centre (0, 0) radius 5.15
  line L0 (-61.64, 2.1) -> (-51.44, 2.1)
  line L1 (-51.44, 2.1) -> (-51.44, -2.1)
  line L2 (-51.44, -2.1) -> (-61.64, -2.1)
  line L3 (-61.64, -2.1) -> (-61.64, 2.1)
  line L4 (-61.64, 2.1) -> (-51.44, -2.1) construction
  line L5 (-51.44, 2.1) -> (-61.64, -2.1) construction
  line L6 (-36.89, 3.1) -> (-26.69, 3.1)
  line L7 (-26.69, 3.1) -> (-26.69, -1.1)
  line L8 (-26.69, -1.1) -> (-36.89, -1.1)
  line L9 (-36.89, -1.1) -> (-36.89, 3.1)
  line L10 (-36.89, 3.1) -> (-26.69, -1.1) construction
  line L11 (-26.69, 3.1) -> (-36.89, -1.1) construction
  line L12 (55.1, 4.1) -> (44.9, 4.1)
  line L13 (44.9, 4.1) -> (44.9, -0.1)
  line L14 (44.9, -0.1) -> (55.1, -0.1)
  line L15 (55.1, -0.1) -> (55.1, 4.1)
  line L16 (55.1, 4.1) -> (44.9, -0.1) construction
  line L17 (44.9, 4.1) -> (55.1, -0.1) construction
  line L18 (105.1, 2.9) -> (94.9, 2.9)
  line L19 (94.9, 2.9) -> (94.9, 7.1)
  line L20 (94.9, 7.1) -> (105.1, 7.1)
  line L21 (105.1, 7.1) -> (105.1, 2.9)
  line L22 (105.1, 2.9) -> (94.9, 7.1) construction
  line L23 (94.9, 2.9) -> (105.1, 7.1) construction
  point P0 (0, 0)
  point P1 (222.2119, -1.834)
  point P2 (221.8244, -1.748)
  point P3 (221.2828, -1.628)
  point P4 (220.5872, -1.4739)
  point P5 (219.7384, -1.287)
  point P6 (218.737, -1.067)
  point P7 (217.5838, -0.8152)
  point P8 (216.2803, -0.532)
  point P9 (214.8275, -0.2185)
  point P10 (213.2266, 0.1249)
  point P11 (211.4794, 0.4969)
  point P12 (209.5871, 0.8964)
  point P13 (207.552, 1.3227)
  point P14 (205.3753, 1.774)
  point P15 (203.0595, 2.2493)
  point P16 (200.607, 2.7475)
  point P17 (198.0195, 3.2675)
  point P18 (195.2996, 3.8074)
  point P19 (192.4502, 4.3658)
  point P20 (189.4737, 4.9416)
  point P21 (186.3728, 5.5333)
  point P22 (183.1508, 6.1395)
  point P23 (179.8104, 6.7584)
  point P24 (176.3554, 7.3885)
  point P25 (172.7881, 8.0288)
  point P26 (169.1129, 8.6773)
  point P27 (165.3325, 9.3327)
  point P28 (161.4514, 9.9931)
  point P29 (157.4723, 10.6576)
  point P30 (153.3999, 11.3241)
  point P31 (149.2378, 11.9914)
  point P32 (144.9901, 12.6578)
  point P33 (140.6608, 13.3221)
  point P34 (136.2544, 13.9826)
  point P35 (131.7746, 14.6376)
  point P36 (127.2264, 15.286)
  point P37 (122.6142, 15.9259)
  point P38 (117.9422, 16.5563)
  point P39 (113.215, 17.1753)
  point P40 (108.4372, 17.7817)
  point P41 (103.6139, 18.3742)
  point P42 (98.7497, 18.9512)
  point P43 (93.8491, 19.511)
  point P44 (88.9175, 20.0526)
  point P45 (83.959, 20.5747)
  point P46 (78.9794, 21.0754)
  point P47 (73.9831, 21.554)
  point P48 (68.9754, 22.0088)
  point P49 (63.9608, 22.439)
  point P50 (58.9451, 22.8427)
  point P51 (53.9326, 23.2187)
  point P52 (48.9288, 23.5667)
  point P53 (43.9384, 23.8847)
  point P54 (38.9668, 24.172)
  point P55 (34.0188, 24.4273)
  point P56 (29.0759, 24.6486)
  point P57 (24.1501, 24.8268)
  point P58 (19.2627, 24.9605)
  point P59 (14.4185, 25.0489)
  point P60 (9.6229, 25.0919)
  point P61 (4.8809, 25.0895)
  point P62 (0.1976, 25.0412)
  point P63 (-4.4224, 24.9478)
  point P64 (-8.9736, 24.8087)
  point P65 (-13.4517, 24.6248)
  point P66 (-17.8516, 24.3963)
  point P67 (-22.1689, 24.1242)
  point P68 (-26.3989, 23.8088)
  point P69 (-30.5374, 23.4512)
  point P70 (-34.5795, 23.0525)
  point P71 (-38.5212, 22.6138)
  point P72 (-42.3587, 22.136)
  point P73 (-46.0874, 21.6211)
  point P74 (-49.7036, 21.0703)
  point P75 (-53.2041, 20.485)
  point P76 (-56.5846, 19.867)
  point P77 (-59.8421, 19.2183)
  point P78 (-62.973, 18.5403)
  point P79 (-65.9744, 17.8348)
  point P80 (-68.8431, 17.1043)
  point P81 (-71.5763, 16.35)
  point P82 (-74.1713, 15.5743)
  point P83 (-76.6261, 14.7792)
  point P84 (-78.9375, 13.9663)
  point P85 (-81.1039, 13.138)
  point P86 (-83.1232, 12.2959)
  point P87 (-84.9934, 11.4418)
  point P88 (-86.7128, 10.5775)
  point P89 (-88.2802, 9.7048)
  point P90 (-89.6939, 8.8255)
  point P91 (-90.9527, 7.9407)
  point P92 (-92.0562, 7.0524)
  point P93 (-93.0026, 6.1611)
  point P94 (-93.792, 5.2685)
  point P95 (-94.4237, 4.3758)
  point P96 (-94.897, 3.4833)
  point P97 (-95.2118, 2.592)
  point P98 (-95.3685, 1.7026)
  point P99 (-95.3665, 0.8156)
  point P100 (-95.2077, -0.0571)
  point P101 (-94.8932, -0.9036)
  point P102 (-94.424, -1.7234)
  point P103 (-93.8007, -2.5165)
  point P104 (-93.0239, -3.2826)
  point P105 (-92.0949, -4.0211)
  point P106 (-91.0147, -4.7323)
  point P107 (-89.7848, -5.4158)
  point P108 (-88.4066, -6.0714)
  point P109 (-86.8815, -6.6986)
  point P110 (-85.2115, -7.2972)
  point P111 (-83.3983, -7.8672)
  point P112 (-81.4439, -8.4081)
  point P113 (-79.3504, -8.9201)
  point P114 (-77.1203, -9.4027)
  point P115 (-74.7554, -9.8562)
  point P116 (-72.2586, -10.28)
  point P117 (-69.6322, -10.6748)
  point P118 (-66.8791, -11.0404)
  point P119 (-64.0017, -11.3765)
  point P120 (-61.0032, -11.6835)
  point P121 (-57.8862, -11.9623)
  point P122 (-54.6543, -12.2122)
  point P123 (-51.3101, -12.4344)
  point P124 (-47.8567, -12.6289)
  point P125 (-44.2979, -12.7967)
  point P126 (-40.6368, -12.9383)
  point P127 (-36.8769, -13.0541)
  point P128 (-33.0214, -13.1455)
  point P129 (-29.0741, -13.2127)
  point P130 (-25.0389, -13.2574)
  point P131 (-20.9193, -13.2799)
  point P132 (-16.7188, -13.2818)
  point P133 (-12.4417, -13.2643)
  point P134 (-8.0914, -13.2281)
  point P135 (-3.6727, -13.175)
  point P136 (0.8111, -13.1058)
  point P137 (5.3558, -13.022)
  point P138 (9.9571, -12.9253)
  point P139 (14.6106, -12.8169)
  point P140 (19.3123, -12.6979)
  point P141 (24.0579, -12.57)
  point P142 (28.843, -12.4341)
  point P143 (33.679, -12.2914)
  point P144 (38.5686, -12.1352)
  point P145 (43.483, -11.9652)
  point P146 (48.4186, -11.7817)
  point P147 (53.3695, -11.5862)
  point P148 (58.3317, -11.38)
  point P149 (63.3002, -11.1641)
  point P150 (68.2698, -10.9392)
  point P151 (73.236, -10.7067)
  point P152 (78.194, -10.4671)
  point P153 (83.139, -10.222)
  point P154 (88.0659, -9.9717)
  point P155 (92.9699, -9.7176)
  point P156 (97.8464, -9.4602)
  point P157 (102.6907, -9.1999)
  point P158 (107.4975, -8.9384)
  point P159 (112.2624, -8.6755)
  point P160 (116.9809, -8.4119)
  point P161 (121.6482, -8.1489)
  point P162 (126.2592, -7.8863)
  point P163 (130.8101, -7.6251)
  point P164 (135.2958, -7.3656)
  point P165 (139.7119, -7.108)
  point P166 (144.0542, -6.853)
  point P167 (148.3186, -6.6011)
  point P168 (152.5, -6.3527)
  point P169 (156.5949, -6.1076)
  point P170 (160.5992, -5.8665)
  point P171 (164.5083, -5.6301)
  point P172 (168.3186, -5.3978)
  point P173 (172.0264, -5.1708)
  point P174 (175.6277, -4.9488)
  point P175 (179.1189, -4.7326)
  point P176 (182.4966, -4.5218)
  point P177 (185.7573, -4.3173)
  point P178 (188.8974, -4.1191)
  point P179 (191.9141, -3.9274)
  point P180 (194.8039, -3.7426)
  point P181 (197.5643, -3.5653)
  point P182 (200.192, -3.3951)
  point P183 (202.6846, -3.233)
  point P184 (205.0394, -3.0789)
  point P185 (207.2539, -2.9329)
  point P186 (209.326, -2.7958)
  point P187 (211.2536, -2.6676)
  point P188 (213.0343, -2.5484)
  point P189 (214.6665, -2.4387)
  point P190 (216.1485, -2.3385)
  point P191 (217.4784, -2.2484)
  point P192 (218.6554, -2.1682)
  point P193 (219.6781, -2.0984)
  point P194 (220.5449, -2.0391)
  point P195 (221.2558, -1.9902)
  point P196 (221.8093, -1.9523)
  point P197 (222.205, -1.9248)
  point P198 (222.4427, -1.9084)
  point P199 (0, 0)
  dimension "d2" = 10.3
  dimension "d38" = 10.2
  dimension "d39" = 4.2
  dimension "d42" = 95.37
  dimension "d43" = -56.54
  dimension "d44" = 0
  dimension "d45" = 10.2
  dimension "d46" = 4.2
  dimension "d128" = 31.79
  dimension "d129" = 1
  dimension "d192" = 10.2
  dimension "d193" = 4.2
  dimension "d196" = 10.2
  dimension "d197" = 4.2
  dimension "d198" = 50
  dimension "d199" = 2
  dimension "d201" = 100
  dimension "d202" = 5
  constraints: 48 end point, 8 midpoint, 8 parallel, 4 horizontal, 4 perpendicular, 1 centre point, 201 other
  measures "d2" diameter of A0
  measures "d38" distance of L1.end L2.end
  measures "d39" distance of L0.end L1.end
  measures "d42" distance of point (-95.367, 0.816) A0.centre
  measures "d43" distance of A0.centre point (-56.54, 0)
  measures "d44" distance of point (0, 0) A0.centre
  measures "d45" distance of L7.end L8.end
  measures "d46" distance of L6.end L7.end
  measures "d128" horizontal distance of point (0, 0) point (-31.79, 1)
  measures "d129" vertical distance of point (0, 0) point (-31.79, 1)
  measures "d192" distance of L14.end L13.end
  measures "d193" distance of L13.end L12.end
  measures "d196" distance of L19.end L20.end
  measures "d197" distance of L18.end L19.end
  measures "d198" horizontal distance of point (0, 0) point (50, 2)
  measures "d199" vertical distance of point (0, 0) point (50, 2)
  measures "d201" horizontal distance of point (100, 5) point (0, 0)
  measures "d202" vertical distance of point (100, 5) point (0, 0)